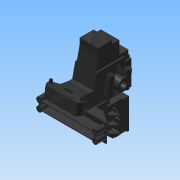
# Autodesk Inventor part: FrontHousing
Saved by Autodesk Inventor 2014 (Build 180170000, 170)
## iProperties
Created: 2014-01-01
Part Number: FrontHousing
Material: ABS Plastic
Document SubType Name: Modeling
Designer: davidgitz
Density: 1.06 g/cm^3
Appearance: Dark Gray
Author: davidgitz
Autodesk Inventor part; units mm, degrees
ref_plane "YZ Plane" through (0, 0, 0) normal (1, 0, 0) x (0, 1, 0)
ref_plane "XZ Plane" through (0, 0, 0) normal (0, 1, 0) x (-1, 0, 0)
ref_plane "XY Plane" through (0, 0, 0) normal (0, 0, 1) x (1, 0, 0)
sketch "Sketch1" plane through (0, 0, 0) normal (1, 0, 0) x (0, 1, 0)
  line L0 (0, 0) -> (-54.0512, 0)
  line L1 (-54.0512, 0) -> (-54.0512, 26.67)
  line L2 (-54.0512, 26.67) -> (-26.6192, 55.88)
  line L3 (-26.6192, 55.88) -> (-26.6192, 69.85)
  line L4 (-26.6192, 69.85) -> (9.4488, 69.85)
  line L5 (9.4488, 69.85) -> (34.4629, 65.4393)
  line L6 (34.4629, 65.4393) -> (34.4629, 58.5813)
  line L7 (34.4629, 58.5813) -> (84.0749, 47.6593)
  line L8 (84.0749, 47.6593) -> (94.2349, 47.6593)
  line L9 (94.2349, 47.6593) -> (94.2349, 23.0213)
  line L10 (94.2349, 23.0213) -> (87.8849, 23.0213)
  line L11 (87.8849, 23.0213) -> (87.8849, 9.8133)
  line L12 (87.8849, 9.8133) -> (65.0249, 9.8133)
  line L13 (65.0249, 9.8133) -> (65.0249, -6.4427)
  line L14 (65.0249, -6.4427) -> (55.6269, -6.4427)
  line L15 (55.6269, -6.4427) -> (55.6269, -8.9827)
  line L16 (55.6269, -8.9827) -> (7.3669, -8.9827)
  line L17 (7.3669, -8.9827) -> (7.3669, 26.5773)
  line L18 (7.3669, 26.5773) -> (0, 26.5773)
  line L19 (0, 26.5773) -> (0, 0)
  dimension "d0" = 54.0512
  dimension "d2" = 26.67
  dimension "d3" = 27.432
  dimension "d4" = 29.21
  dimension "d5" = 13.97
  dimension "d6" = 36.068
  dimension "d9" = 50.8
  dimension "d10" = 10.922
  dimension "d11" = 10.16
  dimension "d12" = 24.638
  dimension "d13" = 6.35
  dimension "d14" = 13.208
  dimension "d15" = 22.86
  dimension "d18" = 16.256
  dimension "d19" = 9.398
  dimension "d20" = 2.54
  dimension "d21" = 48.26
  dimension "d22" = 35.56
  dimension "d23" = 7.3669
  dimension "d24" = 6.858
  dimension "d93" = 10
  dimension "d94" = 86.868
  dimension "d142" = 25.4
  constraints: 40 end point, 15 parallel, 1 coincident, 1 horizontal, 1 perpendicular
  measures "d0" distance of L0.start L0.end
  measures "d2" distance of L0.end L1.end
  measures "d3" distance between parallel lines of L3 L1
  measures "d4" vertical distance of L2.end L1.end
  measures "d5" distance of L2.end L3.end
  measures "d6" distance of L3.end L4.end
  measures "d9" distance of L6.end L7.end
  measures "d10" vertical distance of L7.end L6.end
  measures "d11" distance of L7.end L8.end
  measures "d12" distance of L8.end L9.end
  measures "d13" distance between parallel lines of L9 L11
  measures "d14" distance between parallel lines of L12 L10
  measures "d15" distance between parallel lines of L11 L13
  measures "d18" distance between parallel lines of L12 L14
  measures "d19" distance of L13.end L14.end
  measures "d20" distance between parallel lines of L14 L16
  measures "d21" distance between parallel lines of L15 L17
  measures "d22" distance between parallel lines of L16 L18
  measures "d23" distance between parallel lines of L19 L17
  measures "d24" distance of L5.end L6.end
  measures "d93" angle of L5 L4
  measures "d94" distance between parallel lines of L9 L17
  measures "d142" distance of L4.end L5.end
extrude "Extrusion1" add sketch "Sketch1" along normal mid plane 33.02
sketch "Sketch2" plane through (16.51, 0, 0) normal (1, 0, 0) x (0, 0, -1)
  line L0 (0, -54.0512) -> (0, 0) projected
  line L1 (0, 0) -> (-26.5773, 0) projected
  line L2 (-26.5773, 0) -> (-26.5773, 7.3669) projected
  line L3 (-26.5773, 7.3669) -> (8.9827, 7.3669) projected
  line L4 (8.9827, 7.3669) -> (8.9827, 55.6269) projected
  line L5 (8.9827, 55.6269) -> (6.4427, 55.6269) projected
  line L6 (-47.6593, 84.0749) -> (-58.5813, 34.4629) projected
  line L7 (-58.5813, 34.4629) -> (-65.4393, 34.4629) projected
  line L8 (-65.4393, 34.4629) -> (-69.85, 9.4488) projected
  line L9 (-69.85, 9.4488) -> (-69.85, -26.6192) projected
  line L10 (-69.85, -26.6192) -> (-55.88, -26.6192) projected
  line L11 (-55.88, -26.6192) -> (-26.67, -54.0512) projected
  line L12 (-26.67, -54.0512) -> (0, -54.0512) projected
  line L13 (-53.0834, 59.4369) -> (-1.9393, 59.4369)
  line L14 (-1.9393, 59.4369) -> (-1.9393, 51.8169)
  line L15 (-1.9393, 51.8169) -> (8.9827, 51.8169)
  dimension "d27" = 3.81
  dimension "d28" = 7.62
  dimension "d29" = 10.922
  constraints: 6 end point, 2 perpendicular, 2 point on line, 1 parallel
  measures "d27" distance between parallel lines of L5 L15
  measures "d28" distance of L13.end L14.end
  measures "d29" distance of L14.end L15.end
extrude "Extrusion2" add sketch "Sketch2" along normal blind 2.54
sketch "Sketch3" plane through (19.05, 0, 0) normal (1, 0, 0) x (0, 0, -1)
  line L0 (0, -54.0512) -> (0, 0) projected
  line L1 (0, 0) -> (-26.5773, 0) projected
  line L2 (-69.85, 9.4488) -> (-69.85, -26.6192) projected
  line L3 (-69.85, -26.6192) -> (-55.88, -26.6192) projected
  line L4 (-55.88, -26.6192) -> (-26.67, -54.0512) projected
  line L5 (-26.67, -54.0512) -> (0, -54.0512) projected
  line L6 (-26.5773, 0) -> (-36.7373, 0)
  line L7 (-36.7373, 0) -> (-36.7373, 9.4488)
  line L8 (-36.7373, 9.4488) -> (-69.85, 9.4488)
  dimension "d32" = 10.16
  dimension "d33" = 9.4488
  constraints: 6 end point, 1 horizontal, 1 parallel, 1 vertical
  measures "d32" distance of L1.end L6.end
  measures "d33" distance of L6.end L7.end
extrude "Extrusion3" add sketch "Sketch3" along normal blind 2.54
sketch "Sketch4" plane through (19.05, 0, 0) normal (1, 0, 0) x (0, 0, -1)
  line L0 (-36.7373, 0) -> (-26.5773, 0) projected
  line L1 (-26.5773, 0) -> (-26.5773, 7.3669) projected
  line L2 (-26.5773, 7.3669) -> (8.9827, 7.3669) projected
  arc A0 (-26.5773, 7.3669) -> (-26.5773, 0) centre (-26.5773, 3.6835) ccw
  point P0 (0, 0)
  constraints: 2 point on circle, 2 tangent, 1 centre point
mirror "Mirror1" about plane through (0, 0, 0) normal (1, 0, 0) of "Extrusion2", "Extrusion3"
extrude "Extrusion4" cut sketch "Sketch4" against normal up to next
sketch "Sketch5" plane through (21.59, 0, 0) normal (1, 0, 0) x (0, 0, -1)
  line L0 (0, -54.0512) -> (0, 0) projected
  line L1 (0, 0) -> (-36.7373, 0) projected
  line L2 (-26.67, -54.0512) -> (0, -54.0512) projected
  line L3 (-3.175, -54.0512) -> (-3.175, -3.175)
  line L4 (-3.175, -3.175) -> (-10.16, -3.175)
  line L5 (-10.16, -3.175) -> (-10.16, 0)
  dimension "d38" = 3.175
  dimension "d40" = 3.175
  dimension "d41" = 10.16
  constraints: 6 end point, 3 perpendicular, 2 point on line
  measures "d38" distance of L4.end L5.end
  measures "d40" distance between parallel lines of L0 L3
  measures "d41" distance between parallel lines of L0 L5
extrude "Extrusion5" add sketch "Sketch5" along normal blind 2.54
sketch "Sketch6" plane through (21.59, 0, 0) normal (1, 0, 0) x (0, 0, -1)
  line L0 (0, -54.0512) -> (0, 0) projected
  line L1 (-26.67, -54.0512) -> (0, -54.0512) projected
  line L2 (-26.162, -18.4912) -> (-26.162, -40.3352) construction
  line L3 (-24.892, -37.5644) -> (-24.892, -21.262)
  line L4 (-24.892, -6.0452) -> (-27.432, -6.0452)
  line L5 (-24.892, -15.7204) -> (-24.892, -6.0452)
  arc A0 (-24.892, -21.262) -> (-24.892, -15.7204) centre (-26.162, -18.4912) ccw
  arc A1 (-27.432, -15.7204) -> (-27.432, -21.262) centre (-26.162, -18.4912) ccw
  line L6 (-27.432, -49.7332) -> (-24.892, -49.7332)
  line L7 (-24.892, -49.7332) -> (-24.892, -43.106)
  arc A2 (-24.892, -43.106) -> (-24.892, -37.5644) centre (-26.162, -40.3352) ccw
  line L8 (-27.432, -28.3972) -> (-36.83, -28.3972)
  line L9 (-36.83, -28.3972) -> (-36.83, -25.8572)
  line L10 (-36.83, -25.8572) -> (-27.432, -25.8572)
  line L11 (-27.432, -12.9032) -> (-36.83, -12.9032)
  line L12 (-36.83, -12.9032) -> (-36.83, -10.3632)
  line L13 (-36.83, -10.3632) -> (-27.432, -10.3632)
  line L14 (-27.432, -6.0452) -> (-27.432, -10.3632)
  line L15 (-27.432, -12.9032) -> (-27.432, -15.7204)
  line L16 (-27.432, -37.5644) -> (-27.432, -28.3972)
  line L17 (-27.432, -25.8572) -> (-27.432, -21.262)
  circle A3 centre (-26.162, -18.4912) radius 1.27
  circle A4 centre (-26.162, -40.3352) radius 1.27
  line L18 (-27.432, -43.106) -> (-27.432, -49.7332)
  line L19 (-28.9328, -41.6052) -> (-36.83, -41.6052)
  line L20 (-36.83, -41.6052) -> (-36.83, -39.0652)
  line L21 (-36.83, -39.0652) -> (-28.9328, -39.0652)
  line L22 (-26.162, -40.3352) -> (-28.333, -40.3352) construction
  arc A5 (-27.432, -37.5644) -> (-28.9328, -39.0652) centre (-26.162, -40.3352) ccw
  arc A6 (-28.9328, -41.6052) -> (-27.432, -43.106) centre (-26.162, -40.3352) ccw
  line L23 (-23.5158, -38.8227) -> (-28.8082, -41.8477) construction
  point P0 (-27.432, -32.3463)
  point P1 (-27.432, -22.6709)
  point P2 (-24.892, -32.3463)
  point P3 (-24.892, -22.6709)
  point P4 (-36.83, -40.3352)
  dimension "d47" = 2.54
  dimension "d49" = 4.318
  dimension "d51" = 6.096
  dimension "d52" = 2.54
  dimension "d53" = 8.128
  dimension "d54" = 10.668
  dimension "d55" = 12.954
  dimension "d56" = 43.688
  dimension "d57" = 19.304
  dimension "d58" = 4.318
  dimension "d59" = 24.892
  dimension "d60" = 9.398
  constraints: 44 end point, 14 perpendicular, 12 point on circle, 10 collinear, 8 parallel, 7 centre point, 5 equal radius, 5 point on line, 3 equal length, 2 coincident, 2 midpoint, 2 symmetric about line, 1 horizontal
  measures "d47" distance between parallel lines of L3 L17
  measures "d49" distance between parallel lines of L4 L13
  measures "d51" distance of L23.start L23.end
  measures "d52" diameter of A4
  measures "d53" distance between parallel lines of L19 L6
  measures "d54" distance between parallel lines of L8 L21
  measures "d55" distance between parallel lines of L11 L10
  measures "d56" distance between parallel lines of L6 L4
  measures "d58" distance between parallel lines of L6 L1
  measures "d59" distance between parallel lines of L0 L7
  measures "d60" distance between parallel lines of L12 L14
extrude "Extrusion6" add sketch "Sketch6" along normal blind 11.43
chamfer "Chamfer1" distance 6.35 angle 45 5 edges at (33.02, -40.3352, 36.83) (33.02, -27.1272, 36.83) (33.02, -11.6332, 36.83) (33.02, -49.7332, 26.162) (33.02, -6.0452, 26.162)
mirror "Mirror2" about plane through (0, 0, 0) normal (1, 0, 0) of "Extrusion5", "Extrusion6", "Chamfer1"
sketch "Sketch7" plane through (-19.05, 7.3669, -8.9827) normal (-1, 0, 0) x (0, 0, 1)
  line L0 (0, 0) -> (0, 44.45) projected
  line L1 (35.56, 0) -> (0, 0) projected
  circle A0 centre (26.924, 23.368) radius 10.414
  line L2 (16.51, 32.9979) -> (16.51, 6.5502) construction
  line L3 (5.461, 12.954) -> (33.4427, 12.954) construction
  circle A1 centre (26.924, 23.368) radius 5.842
  point P0 (8.9827, -7.3669)
  dimension "d67" = 20.828
  dimension "d69" = 12.954
  dimension "d70" = 16.51
  dimension "d72" = 11.684
  constraints: 4 end point, 2 centre point, 2 coincident, 2 perpendicular, 2 tangent
  measures "d67" diameter of A0
  measures "d69" distance between parallel lines of L1 L3
  measures "d70" distance between parallel lines of L2 L0
  measures "d72" diameter of A1
extrude "Extrusion7" add sketch "Sketch7" along normal blind 13.716
sketch "Sketch8" plane through (-19.05, 7.3669, -8.9827) normal (-1, 0, 0) x (0, 0, 1)
  line L0 (0, 0) -> (0, 44.45) projected
  circle A0 centre (26.924, 23.368) radius 10.414 projected
  line L1 (23.6237, 42.0847) -> (30.2243, 4.6513) construction
  line L2 (44.4492, 41.2885) -> (34.8938, 39.6036)
  line L3 (34.8938, 39.6036) -> (39.9661, 10.8374)
  line L4 (39.9661, 10.8374) -> (49.5215, 12.5222)
  line L5 (49.5215, 12.5222) -> (44.4492, 41.2885)
  line L6 (24.4918, 44.4753) -> (23.2411, 44.2548)
  line L7 (24.4918, 44.4753) -> (26.3798, 33.7678)
  line L8 (26.924, 23.368) -> (33.1614, 24.4678) construction
  line L9 (31.8576, 2.7017) -> (30.6069, 2.4812)
  line L10 (31.8576, 2.7017) -> (29.9696, 13.4093)
  line L11 (4.3265, 34.2138) -> (13.8819, 35.8986)
  line L12 (13.8819, 35.8986) -> (18.9542, 7.1324)
  line L13 (18.9542, 7.1324) -> (9.3988, 5.4475)
  line L14 (9.3988, 5.4475) -> (4.3265, 34.2138)
  line L15 (21.9904, 44.0343) -> (23.2411, 44.2548)
  line L16 (21.9904, 44.0343) -> (23.8784, 33.3267)
  line L17 (29.3562, 2.2607) -> (30.6069, 2.4812)
  line L18 (29.3562, 2.2607) -> (27.4682, 12.9682)
  arc A1 (27.4682, 12.9682) -> (29.9696, 13.4093) centre (26.924, 23.368) ccw
  arc A2 (26.3798, 33.7678) -> (23.8784, 33.3267) centre (26.924, 23.368) ccw
  point P0 (8.9827, -7.3669)
  point P1 (37.4299, 25.2205)
  dimension "d75" = 10
  dimension "d76" = 9.7028
  dimension "d78" = 6.604
  dimension "d79" = 29.21
  dimension "d80" = 9.398
  dimension "d81" = 2.54
  constraints: 36 end point, 11 symmetric about line, 4 perpendicular, 4 point on circle, 3 parallel, 2 centre point, 2 coincident, 2 midpoint, 2 point on line, 2 other
  measures "d75" angle of L0 L1
  measures "d76" distance between parallel lines of L3 L5
  measures "d78" distance between parallel lines of L2 L6
  measures "d79" distance between parallel lines of L4 L2
  measures "d80" distance between parallel lines of L7 L3
  measures "d81" distance between parallel lines of L16 L7
extrude "Extrusion8" add sketch "Sketch8" along normal blind 8.89 contours A0 L16 L15 L6 L7 | L10 L9 L17 L18 A0 | L5 L4 L3 L2 | L11 L12 L13 L14
chamfer "Chamfer2" distance 6.35 angle 45 2 edges at (-27.94, 51.6217, 14.2584) (-27.94, 9.8481, 21.6242)
sketch "Sketch9" plane through (-27.94, 46.9705, 25.9111) normal (0, 0.9848078, -0.1736482) x (1, 0, 0)
  line L0 (8.89, 0) -> (8.89, -9.7028) projected
  line L1 (8.89, 0) -> (0, 0) projected
  circle A0 centre (4.8514, -4.8514) radius 1.5875
  arc A1 (0, -4.8514) -> (4.8514, -9.7028) centre (4.8514, -4.8514) ccw
  line L2 (0, -9.7028) -> (4.8514, -9.7028)
  line L3 (0, -9.7028) -> (0, -4.8514)
  line L4 (4.8514, -4.8514) -> (-6.5715, -4.8514) construction
  arc A2 (4.8514, 0) -> (0, -4.8514) centre (4.8514, -4.8514) ccw
  line L5 (0, 0) -> (4.8514, 0)
  line L6 (0, 0) -> (0, -4.8514)
  point P0 (27.94, 33.6738)
  dimension "d87" = 3.175
  constraints: 11 end point, 4 point on circle, 3 centre point, 3 symmetric about line, 2 coincident, 2 point on line, 1 perpendicular, 1 tangent, 1 other
  measures "d87" diameter of A0
extrude "Extrusion9" cut sketch "Sketch9" against normal up to next
ref_plane "Work Plane2" through (-19.05, 30.7349, 17.9413) normal (0, 0.1736482, 0.9848078) x (-1, 0, 0)
mirror "Mirror3" about plane through (-19.05, 30.7349, 17.9413) normal (0, 0.1736482, 0.9848078) of "Extrusion9"
mirror "Mirror4" about plane through (0, 0, 0) normal (1, 0, 0) of "Extrusion7", "Extrusion8", "Chamfer2", "Extrusion9", "Mirror3"
ref_plane "Work Plane3" through (0, 34.4629, 65.4393) normal (0, 0.9848078, -0.1736482) x (-1, 0, 0)
sketch "Sketch10" plane through (0, 34.4629, 65.4393) normal (0, 0.9848078, -0.1736482) x (-1, 0, 0)
  line L0 (-19.05, 0) -> (19.05, 0) projected
  line L1 (19.05, 0) -> (19.05, -32.6096) projected
  line L2 (21.59, -32.6096) -> (21.59, 0) projected
  line L3 (19.05, 0) -> (19.05, 12.6773)
  line L4 (20.9243, 15.5737) -> (29.559, 19.4512)
  line L5 (31.7674, 25.6823) -> (29.3285, 30.5138)
  line L6 (26.4942, 32.258) -> (0, 32.258)
  arc A0 (29.559, 19.4512) -> (31.7674, 25.6823) centre (27.686, 23.622) ccw
  line L7 (32.258, 30.6365) -> (32.258, 14.3925) construction
  line L8 (0, 0) -> (0, 37.5619) construction
  arc A1 (29.3285, 30.5138) -> (26.4942, 32.258) centre (26.4942, 29.083) ccw
  arc A2 (20.9243, 15.5737) -> (19.05, 12.6773) centre (22.225, 12.6773) ccw
  line L9 (0, 21.2852) -> (7.5311, 21.2852)
  line L10 (7.5311, 21.2852) -> (7.5311, 15.24)
  line L11 (7.5311, 15.24) -> (0, 15.24)
  line L12 (-19.05, 0) -> (-19.05, 12.6773)
  line L13 (-20.9243, 15.5737) -> (-29.559, 19.4512)
  line L14 (-31.7674, 25.6823) -> (-29.3285, 30.5138)
  line L15 (-26.4942, 32.258) -> (0, 32.258)
  arc A3 (-31.7674, 25.6823) -> (-29.559, 19.4512) centre (-27.686, 23.622) ccw
  line L16 (-32.258, 30.6365) -> (-32.258, 14.3925) construction
  arc A4 (-26.4942, 32.258) -> (-29.3285, 30.5138) centre (-26.4942, 29.083) ccw
  arc A5 (-19.05, 12.6773) -> (-20.9243, 15.5737) centre (-22.225, 12.6773) ccw
  line L17 (0, 21.2852) -> (-7.5311, 21.2852)
  line L18 (-7.5311, 21.2852) -> (-7.5311, 15.24)
  line L19 (-7.5311, 15.24) -> (0, 15.24)
  point P0 (0, -70.4296)
  point P1 (19.05, -33.0808)
  point P2 (21.59, -33.0808)
  point P3 (19.05, 14.732)
  point P4 (28.448, 32.258)
  point P5 (-21.59, 0)
  point P6 (-19.05, 14.732)
  point P7 (-28.448, 32.258)
  dimension "d96" = 14.732
  dimension "d97" = 13.208
  dimension "d99" = 17.526
  dimension "d101" = 3.81
  dimension "d102" = 8.636
  dimension "d103" = 4.572
  dimension "d104" = 3.175
  dimension "d105" = 10.9728
  dimension "d106" = 6.0452
  dimension "d108" = 15.0622
  constraints: 34 end point, 16 symmetric about line, 12 point on circle, 11 point on line, 7 tangent, 6 centre point, 4 perpendicular, 2 parallel, 1 equal radius, 1 midpoint, 1 vertical, 3 other
  measures "d96" distance of L0.end point (19.05, 14.732)
  measures "d97" distance between parallel lines of L3 L7
  measures "d99" distance from line of point (19.05, 14.732) L6
  measures "d101" distance from line of L7 point (28.448, 32.258)
  measures "d102" distance from line of A0.centre L6
  measures "d103" distance from line of L7 A0.centre
  measures "d104" radius of A1
  measures "d105" distance between parallel lines of L6 L9
  measures "d106" distance of L9.end L10.end
  measures "d108" distance between parallel lines of L18 L10
extrude "Extrusion10" add sketch "Sketch10" against normal blind 19.4818
sketch "Sketch11" plane through (0, 34.4629, 65.4393) normal (0, 0.9848078, -0.1736482) x (1, 0, 0)
  line L0 (19.05, 0) -> (-19.05, 0) projected
  arc A0 (-29.559, -19.4512) -> (-31.7674, -25.6823) centre (-27.686, -23.622) ccw projected
  line L1 (19.05, -12.6773) -> (19.05, 0) projected
  circle A1 centre (-27.686, -23.622) radius 2.4638
  circle A2 centre (-27.686, -23.622) radius 1.27
  line L2 (0, 0) -> (0, -35.4609) construction
  circle A3 centre (27.686, -23.622) radius 2.4638
  circle A4 centre (27.686, -23.622) radius 1.27
  point P0 (0, 70.4296)
  dimension "d111" = 4.9276
  dimension "d112" = 2.54
  constraints: 4 centre point, 4 coincident, 3 symmetric about line, 2 end point, 1 midpoint, 1 parallel, 2 other
  measures "d111" diameter of A1
  measures "d112" diameter of A2
extrude "Extrusion11" add sketch "Sketch11" along normal blind 5.461
sketch "Sketch12" plane through (19.05, 9.4488, 69.85) normal (0, 0, 1) x (1, 0, 0)
  line L0 (2.54, -36.068) -> (-40.64, -36.068) projected
  line L1 (0, 0) -> (-38.1, 0) projected
  line L2 (-73.8378, -32.766) -> (35.7378, -32.766)
  line L3 (35.7378, -32.766) -> (35.7378, 0)
  line L4 (35.7378, 0) -> (-73.8378, 0)
  line L5 (-73.8378, 0) -> (-73.8378, -32.766)
  line L6 (-19.05, 0) -> (-19.05, -94.8078) construction
  point P0 (-19.05, -9.4488)
  point P1 (-19.05, -36.068)
  dimension "d115" = 109.5756
  dimension "d116" = 32.766
  constraints: 10 end point, 3 midpoint, 3 point on line, 2 parallel, 1 horizontal, 1 perpendicular
  measures "d115" distance of L2.start L2.end
  measures "d116" distance of L2.end L3.end
extrude "Extrusion12" add sketch "Sketch12" along normal blind 2.032
sketch "Sketch13" plane through (-54.7878, -23.3172, 69.85) normal (0, -1, 0) x (1, 0, 0)
  line L0 (76.3778, 0) -> (109.5756, 0) projected
  line L1 (76.3778, 0) -> (76.3778, -13.97) projected
  line L2 (109.5756, 0) -> (89.0778, -13.97)
  line L3 (89.0778, -13.97) -> (76.3778, -13.97)
  line L4 (76.3778, -13.97) -> (76.3778, 0)
  line L5 (76.3778, 0) -> (109.5756, 0)
  point P0 (54.7878, -69.85)
  dimension "d120" = 12.7
  constraints: 8 end point, 2 collinear, 1 horizontal
  measures "d120" distance of L2.end L1.end
extrude "Extrusion13" add sketch "Sketch13" against normal up to surface (32.766 mm away)
sketch "Sketch14" plane through (54.7878, -23.3172, 71.882) normal (1, 0, 0) x (0, 0, -1)
  line L0 (2.032, 0) -> (2.032, 32.766) projected
  line L1 (16.002, 32.766) -> (2.032, 32.766) projected
  line L2 (2.032, 0) -> (2.032, 32.766) projected
  line L3 (16.002, 0) -> (2.032, 0) projected
  line L4 (16.002, 0) -> (16.002, 32.766) projected
  line L5 (2.032, 30.226) -> (16.002, 30.226)
  line L6 (16.002, 30.226) -> (16.002, 2.54)
  line L7 (16.002, 2.54) -> (2.032, 2.54)
  line L8 (2.032, 2.54) -> (2.032, 30.226)
  point P0 (71.882, 23.3172)
  dimension "d123" = 2.54
  dimension "d124" = 2.54
  constraints: 8 end point, 2 parallel, 2 point on line, 1 horizontal, 1 perpendicular
  measures "d123" distance between parallel lines of L1 L5
  measures "d124" distance between parallel lines of L3 L7
extrude "Extrusion14" cut sketch "Sketch14" against normal up to surface (33.1978 mm away) contours L0 L5 L4 L7
mirror "Mirror5" about plane through (0, 0, 0) normal (1, 0, 0) of "Extrusion13", "Extrusion14"
sketch "Sketch15" plane through (19.05, 9.4488, 71.882) normal (0, 0, 1) x (1, 0, 0)
  line L0 (-73.8378, -32.766) -> (35.7378, -32.766) projected
  line L1 (35.7378, -32.766) -> (35.7378, 0) projected
  line L2 (35.7378, 0) -> (-73.8378, 0) projected
  line L3 (-19.05, 0) -> (-19.05, -32.766) construction
  line L4 (30.9753, -9.2075) -> (30.9753, -23.5585) construction
  line L5 (14.9638, -28.321) -> (43.1136, -28.321) construction
  line L6 (12.4502, -4.445) -> (40.8538, -4.445) construction
  arc A0 (26.2553, -9.8425) -> (30.3403, -13.9275) centre (30.9753, -9.2075) ccw
  line L7 (30.9753, -9.2075) -> (-5.2173, -9.2075) construction
  line L8 (35.7378, -16.383) -> (12.879, -16.383) construction
  line L9 (30.3403, -13.9275) -> (30.3403, -16.383)
  line L10 (31.6103, -13.9275) -> (31.6103, -16.383)
  line L11 (26.2553, -8.5725) -> (-19.05, -8.5725)
  line L12 (26.2553, -9.8425) -> (-19.05, -9.8425)
  arc A1 (31.6103, -13.9275) -> (26.2553, -8.5725) centre (30.9753, -9.2075) ccw
  arc A2 (26.2553, -9.8425) -> (30.3403, -13.9275) centre (30.9753, -9.2075) ccw
  circle A3 centre (30.9753, -9.2075) radius 1.5875
  arc A4 (30.3403, -18.8385) -> (26.2553, -22.9235) centre (30.9753, -23.5585) ccw
  line L13 (30.3403, -18.8385) -> (30.3403, -16.383)
  line L14 (31.6103, -18.8385) -> (31.6103, -16.383)
  line L15 (26.2553, -24.1935) -> (-19.05, -24.1935)
  line L16 (26.2553, -22.9235) -> (-19.05, -22.9235)
  arc A5 (26.2553, -24.1935) -> (31.6103, -18.8385) centre (30.9753, -23.5585) ccw
  circle A6 centre (30.9753, -23.5585) radius 1.5875
  line L17 (-73.8378, -32.766) -> (-73.8378, 0)
  line L18 (-69.0753, -9.2075) -> (-69.0753, -23.5585) construction
  line L19 (-53.0638, -28.321) -> (-81.2136, -28.321) construction
  line L20 (-50.5502, -4.445) -> (-78.9538, -4.445) construction
  arc A7 (-68.4403, -13.9275) -> (-64.3553, -9.8425) centre (-69.0753, -9.2075) ccw
  line L21 (-69.0753, -9.2075) -> (-32.8827, -9.2075) construction
  line L22 (-73.8378, -16.383) -> (-50.979, -16.383) construction
  line L23 (-68.4403, -13.9275) -> (-68.4403, -16.383)
  line L24 (-69.7103, -13.9275) -> (-69.7103, -16.383)
  line L25 (-64.3553, -8.5725) -> (-19.05, -8.5725)
  line L26 (-64.3553, -9.8425) -> (-19.05, -9.8425)
  arc A8 (-64.3553, -8.5725) -> (-69.7103, -13.9275) centre (-69.0753, -9.2075) ccw
  arc A9 (-68.4403, -13.9275) -> (-64.3553, -9.8425) centre (-69.0753, -9.2075) ccw
  circle A10 centre (-69.0753, -9.2075) radius 1.5875
  line L27 (-64.3553, -24.1935) -> (-19.05, -24.1935)
  line L28 (-64.3553, -22.9235) -> (-19.05, -22.9235)
  arc A11 (-69.7103, -18.8385) -> (-64.3553, -24.1935) centre (-69.0753, -23.5585) ccw
  arc A12 (-64.3553, -22.9235) -> (-68.4403, -18.8385) centre (-69.0753, -23.5585) ccw
  circle A13 centre (-69.0753, -23.5585) radius 1.5875
  line L29 (-69.7103, -18.8385) -> (-69.7103, -16.383)
  line L30 (-68.4403, -18.8385) -> (-68.4403, -16.383)
  point P0 (-19.05, -9.4488)
  point P1 (30.9753, -16.383)
  point P2 (-69.0753, -16.383)
  dimension "d130" = 4.445
  dimension "d131" = 4.445
  dimension "d137" = 0.635
  dimension "d138" = 0.635
  dimension "d139" = 3.175
  constraints: 56 end point, 29 symmetric about line, 20 point on circle, 14 centre point, 5 parallel, 4 coincident, 4 midpoint, 3 horizontal, 3 perpendicular, 2 point on line, 2 tangent, 1 vertical, 10 other
  measures "d130" distance between parallel lines of L0 L5
  measures "d131" distance between parallel lines of L2 L6
  measures "d137" distance between parallel lines of L4 L10
  measures "d138" distance between parallel lines of L7 L11
  measures "d139" diameter of A3
ref_plane "Work Plane4" through (-55.118, 276.099, 82.677) normal (0, 0, 1) x (1, 0, 0)
extrude "Extrusion15" add sketch "Sketch15" along normal blind 15.4686 contours A11 L29 L24 A8 L25 L11 A1 L10 L14 A5 L15 L27
body "Solid1"
